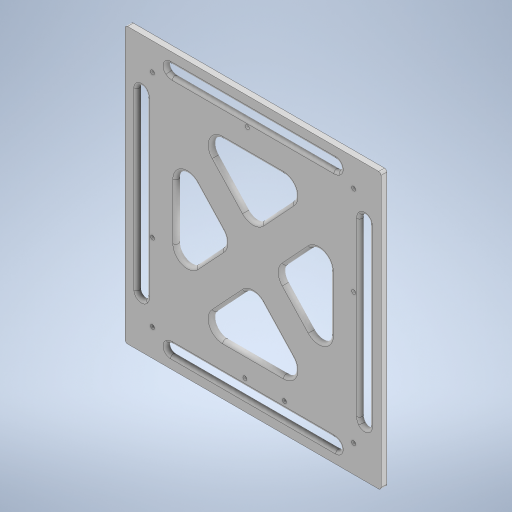
# Autodesk Inventor part: LI0009 XILINX SHELF
Saved by Autodesk Inventor 2023 (Build 270158000, 158)
## iProperties
Created: 2023-04-03
Part Number: LI0009 XILINX SHELF
Material: Generic
Document SubType Name: Modeling
Designer: Louis
Density: 1 g/cm^3
Appearance: Default
Author: Louis
Autodesk Inventor part; units mm, degrees
ref_plane "YZ Plane" through (0, 0, 0) normal (1, 0, 0) x (0, 1, 0)
ref_plane "XZ Plane" through (0, 0, 0) normal (0, 1, 0) x (-1, 0, 0)
ref_plane "XY Plane" through (0, 0, 0) normal (0, 0, 1) x (1, 0, 0)
sketch "Sketch1" plane through (0, 0, 0) normal (0, 0, 1) x (1, 0, 0)
  line L0 (-110, 118.25) -> (110, 118.25)
  line L1 (110, 118.25) -> (110, -118.25)
  line L2 (110, -118.25) -> (-110, -118.25)
  line L3 (-110, -118.25) -> (-110, 118.25)
  point P0 (0, 0)
  point P1 (0, 118.25)
  point P2 (-110, 0)
  dimension "d1" = 220
  dimension "d2" = 236.5
  constraints: 8 end point, 2 midpoint, 2 parallel, 1 horizontal, 1 horizontal alignment, 1 perpendicular, 1 vertical alignment
  measures "d1" distance of L0.start L0.end
  measures "d2" distance of L0.end L1.end
extrude "Extrusion1" add sketch "Sketch1" along normal blind 5
sketch "Sketch2" plane through (0, 0, 5) normal (0, 0, 1) x (1, 0, 0)
  line L0 (-90, 98.25) -> (90, 98.25)
  line L1 (90, 98.25) -> (90, -98.25)
  line L2 (90, -98.25) -> (-90, -98.25)
  line L3 (-90, -98.25) -> (-90, 98.25)
  line L4 (-86.5, 94.75) -> (86.5, 94.75)
  line L5 (86.5, 94.75) -> (86.5, -94.75)
  line L6 (86.5, -94.75) -> (-86.5, -94.75)
  line L7 (-86.5, -94.75) -> (-86.5, 94.75)
  line L8 (-6.99, -93.25) -> (27, -93.25)
  point P0 (0, 0)
  point P1 (0, 98.25)
  point P2 (-90, 0)
  point P3 (-86.5, -28.25)
  point P4 (86.5, 17.75)
  point P5 (-5, 94.75)
  dimension "d5" = 180
  dimension "d6" = 196.5
  dimension "d7" = 3.5
  dimension "d8" = 3.5
  dimension "d10" = 3.5
  dimension "d11" = 3.5
  dimension "d12" = 70
  dimension "d13" = 116
  dimension "d16" = 85
  dimension "d24" = 83.01
  dimension "d25" = 117
  dimension "d26" = 5
  constraints: 18 end point, 6 coincident, 4 parallel, 3 horizontal, 3 point on line, 2 midpoint, 2 perpendicular, 1 horizontal alignment, 1 vertical alignment
  measures "d5" distance of L0.start L0.end
  measures "d6" distance of L2.end L0.start
  measures "d7" distance between parallel lines of L2 L6
  measures "d8" distance between parallel lines of L3 L7
  measures "d10" distance between parallel lines of L0 L4
  measures "d11" distance between parallel lines of L1 L5
  measures "d12" distance from line of L2 point (-86.5, -28.25)
  measures "d13" distance from line of L2 point (86.5, 17.75)
  measures "d16" distance from line of L3 point (-5, 94.75)
  measures "d24" distance from line of L3 L8.start
  measures "d25" distance from line of L3 L8.end
  measures "d26" distance between parallel lines of L2 L8
hole "Hole1" at (-86.5, -94.75, 5) at (86.5, -94.75, 5) at (-86.5, 94.75, 5) at (86.5, 94.75, 5) at (-86.5, -28.25, 5) at (86.5, 17.75, 5) at (-5, 94.75, 5) at (-6.99, -93.25, 5) at (27, -93.25, 5) direction (0, 0, -1) diameter 3.4 end through all clearance for "Flat Head Machine Screw" size "M3" standard "Ansi Metric M Profile"
sketch "Sketch3" plane through (0, 0, 5) normal (0, 0, 1) x (1, 0, 0)
  circle A0 centre (-86.5, 94.75) radius 1.7 projected
  circle A1 centre (86.5, -94.75) radius 1.7 projected
  line L0 (-86.5, 94.75) -> (86.5, 94.75)
  line L1 (86.5, 94.75) -> (86.5, -94.75)
  line L2 (86.5, -94.75) -> (-86.5, -94.75)
  line L3 (-86.5, -94.75) -> (-86.5, 94.75)
  line L4 (-110, 118.25) -> (-110, -118.25) projected
  line L5 (110, 118.25) -> (-110, 118.25) projected
  line L6 (110, -118.25) -> (110, 118.25) projected
  line L7 (-110, -118.25) -> (110, -118.25) projected
  line L8 (-100, 108.25) -> (-100, -108.25)
  line L9 (-100, -108.25) -> (100, -108.25)
  line L10 (100, -108.25) -> (100, 108.25)
  line L11 (100, 108.25) -> (-100, 108.25)
  line L12 (91.5, 99.75) -> (-91.5, 99.75)
  line L13 (-91.5, 99.75) -> (-91.5, -99.75)
  line L14 (-91.5, -99.75) -> (91.5, -99.75)
  line L15 (91.5, -99.75) -> (91.5, 99.75)
  line L16 (66.5, 74.75) -> (-66.5, 74.75)
  line L17 (-66.5, 74.75) -> (-66.5, -74.75)
  line L18 (-66.5, -74.75) -> (66.5, -74.75)
  line L19 (66.5, -74.75) -> (66.5, 74.75)
  line L20 (-110, 118.25) -> (-110, -118.25) projected
  line L21 (-110, 118.25) -> (110, -118.25)
  line L22 (110, 118.25) -> (-110, -118.25)
  line L23 (99.0172, 128.4666) -> (-120.9828, -108.0334)
  line L24 (120.9828, 108.0334) -> (-99.0172, -128.4666)
  line L25 (-120.9828, 108.0334) -> (99.0172, -128.4666)
  line L26 (-99.0172, 128.4666) -> (120.9828, -108.0334)
  point P0 (0, 0)
  point P1 (91.5, -76.3394)
  point P2 (100, -85.4769)
  point P3 (100, 85.4769)
  point P4 (91.5, 76.3394)
  point P5 (80.2111, -108.25)
  point P6 (72.3041, -99.75)
  point P7 (-72.3041, -99.75)
  point P8 (-80.2111, -108.25)
  point P9 (-91.5, 76.3394)
  point P10 (-100, 85.4769)
  point P11 (-100, -85.4769)
  point P12 (-91.5, -76.3394)
  point P13 (-80.2111, 108.25)
  point P14 (-72.3041, 99.75)
  point P15 (72.3041, 99.75)
  point P16 (80.2111, 108.25)
  point P17 (49.0483, -74.75)
  point P18 (0, -22.0231)
  point P19 (-49.0483, -74.75)
  point P20 (20.4866, 0)
  point P21 (66.5, -49.4644)
  point P22 (66.5, 49.4644)
  point P23 (-49.0483, 74.75)
  point P24 (0, 22.0231)
  point P25 (49.0483, 74.75)
  point P26 (-20.4866, 0)
  point P27 (-66.5, 49.4644)
  point P28 (-66.5, -49.4644)
  dimension "d27" = 10
  dimension "d28" = 5
  dimension "d29" = 20
  dimension "d30" = 15
  dimension "d31" = 15
  dimension "d32" = 15
  dimension "d33" = 15
  constraints: 44 end point, 10 parallel, 3 perpendicular, 1 horizontal, 9 other
  measures "d27" distance between parallel lines of L5 L11
  measures "d28" distance between parallel lines of L0 L12
  measures "d29" distance between parallel lines of L0 L16
  measures "d30" distance between parallel lines of L22 L23
  measures "d31" distance between parallel lines of L22 L24
  measures "d32" distance between parallel lines of L21 L25
  measures "d33" distance between parallel lines of L21 L26
extrude "Extrusion2" cut sketch "Sketch3" against normal through all contours L26 L11 L23 L12 | L16 L23 L26 | L13 L23 L8 L25 | L25 L23 L17 | L24 L19 L26 | L24 L10 L26 L15 | L14 L25 L9 L24 | L25 L18 L24
fillet "Fillet1" radius 10 12 edges at (0, 22.0231, 2.5) (-49.0483, 74.75, 2.5) (49.0483, 74.75, 2.5) (66.5, 49.4644, 2.5) (20.4866, 0, 2.5) (66.5, -49.4644, 2.5) (49.0483, -74.75, 2.5) (0, -22.0231, 2.5) (-49.0483, -74.75, 2.5) (-66.5, -49.4644, 2.5) (-20.4866, 0, 2.5) (-66.5, 49.4644, 2.5)
fillet "Fillet2" radius 6.5 8 edges at (91.5, 76.3394, 2.5) (91.5, -76.3394, 2.5) (72.3041, -99.75, 2.5) (-72.3041, -99.75, 2.5) (-91.5, -76.3394, 2.5) (-91.5, 76.3394, 2.5) (-72.3041, 99.75, 2.5) (72.3041, 99.75, 2.5)
fillet "Fillet3" radius 2 4 edges at (110, 118.25, 2.5) (110, -118.25, 2.5) (-110, -118.25, 2.5) (-110, 118.25, 2.5)
fillet "Fillet6" radius 4 8 edges at (-100, 85.4769, 2.5) (-80.2111, 108.25, 2.5) (80.2111, 108.25, 2.5) (100, 85.4769, 2.5) (100, -85.4769, 2.5) (80.2111, -108.25, 2.5) (-80.2111, -108.25, 2.5) (-100, -85.4769, 2.5)
fillet "Fillet7" radius 2.5 96 edges at (-97.2649, 79.0783, 5) (-91.8336, 75.8391, 5) (-91.5, 0, 5) (-91.8336, -75.8391, 5) (-97.2649, -79.0783, 5) (-100, 0, 5) (-60.1593, 33.3388, 5) (-38.0003, 18.8272, 5) (-24.1443, 0, 5) (-38.0003, -18.8272, 5) (-60.1593, -33.3388, 5) (-66.5, 0, 5) (35.2564, 68.7431, 5) (20.366, 43.9165, 5) (0, 26.7051, 5) (-20.366, 43.9165, 5) (-35.2564, 68.7431, 5) (0, 74.75, 5) (38.0003, -18.8272, 5) (60.1593, -33.3388, 5) (66.5, 0, 5) (60.1593, 33.3388, 5) (38.0003, 18.8272, 5) (24.1443, 0, 5) (35.2564, -68.7431, 5) (0, -74.75, 5) (-35.2564, -68.7431, 5) (-20.366, -43.9165, 5) (0, -26.7051, 5) (20.366, -43.9165, 5) (91.8336, 75.8391, 5) (97.2649, 79.0783, 5) (100, 0, 5) (97.2649, -79.0783, 5) (91.8336, -75.8391, 5) (91.5, 0, 5) (71.5286, -100.0836, 5) (74.7678, -105.5149, 5) (0, -108.25, 5) (-74.7678, -105.5149, 5) (-71.5286, -100.0836, 5) (0, -99.75, 5) (-71.5286, 100.0836, 5) (-74.7678, 105.5149, 5) (0, 108.25, 5) (74.7678, 105.5149, 5) (71.5286, 100.0836, 5) (0, 99.75, 5) (97.2649, 79.0783, 0) (91.8336, 75.8391, 0) (91.5, 0, 0) (91.8336, -75.8391, 0) (97.2649, -79.0783, 0) (100, 0, 0) (-74.7678, 105.5149, 0) (-71.5286, 100.0836, 0) (0, 99.75, 0) (71.5286, 100.0836, 0) (74.7678, 105.5149, 0) (0, 108.25, 0) (35.2564, 68.7431, 0) (0, 74.75, 0) (-35.2564, 68.7431, 0) (-20.366, 43.9165, 0) (0, 26.7051, 0) (20.366, 43.9165, 0) (24.1443, 0, 0) (38.0003, -18.8272, 0) (60.1593, -33.3388, 0) (66.5, 0, 0) (60.1593, 33.3388, 0) (38.0003, 18.8272, 0) (-60.1593, 33.3388, 0) (-66.5, 0, 0) (-60.1593, -33.3388, 0) (-38.0003, -18.8272, 0) (-24.1443, 0, 0) (-38.0003, 18.8272, 0) (-35.2564, -68.7431, 0) (0, -74.75, 0) (35.2564, -68.7431, 0) (20.366, -43.9165, 0) (0, -26.7051, 0) (-20.366, -43.9165, 0) (-91.8336, 75.8391, 0) (-97.2649, 79.0783, 0) (-100, 0, 0) (-97.2649, -79.0783, 0) (-91.8336, -75.8391, 0) (-91.5, 0, 0) (-71.5286, -100.0836, 0) (-74.7678, -105.5149, 0) (0, -108.25, 0) (74.7678, -105.5149, 0) (71.5286, -100.0836, 0) (0, -99.75, 0)
body "Solid1"
